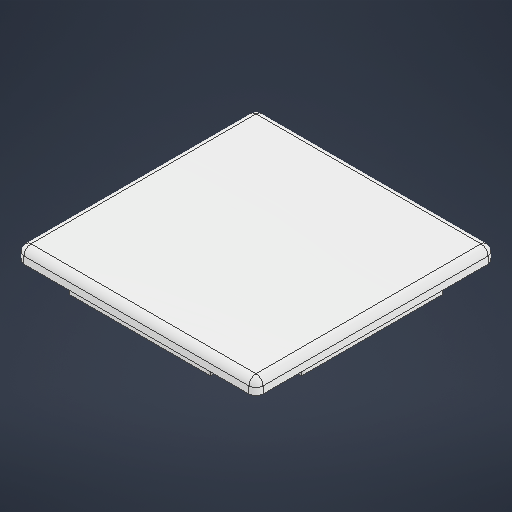
# Autodesk Inventor part: block_main
Saved by Autodesk Inventor 2025.2 (Build 292293000, 293)
## iProperties
Created: 2025-08-04
Part Number: block_main
Material: PC/ABS Plastic
Document SubType Name: Modeling
Designer: sam
Density: 1.1 g/cm^3
Appearance: Smooth - White
Author: sam
Autodesk Inventor part; units mm, degrees
ref_plane "YZ Plane" through (0, 0, 0) normal (1, 0, 0) x (0, 1, 0)
ref_plane "XZ Plane" through (0, 0, 0) normal (0, 1, 0) x (-1, 0, 0)
ref_plane "XY Plane" through (0, 0, 0) normal (0, 0, 1) x (1, 0, 0)
sketch "Sketch4" plane through (0, 0, 0) normal (0, 1, 0) x (-1, 0, 0)
  line L0 (17, 17) -> (-17, 17)
  line L1 (-17, 17) -> (-17, -17)
  line L2 (-17, -17) -> (17, -17)
  line L3 (17, -17) -> (17, 17)
  line L4 (17, 17) -> (-17, -17) construction
  line L5 (-17, 17) -> (17, -17) construction
  point P0 (0, 0)
  dimension "d52" = 34
  dimension "d53" = 34
  constraints: 12 end point, 2 midpoint, 2 parallel, 1 horizontal, 1 perpendicular
  measures "d52" distance of L2.end L1.end
  measures "d53" distance of L1.end L0.end
extrude "Extrusion5" add sketch "Sketch4" along normal blind 2
sketch "Sketch6" plane through (0, 0, 0) normal (0, -1, 0) x (1, 0, 0)
  line L0 (-16.5, -10) -> (-15.5, -10)
  line L1 (-15.5, -10) -> (-15.5, 10)
  line L2 (-15.5, 10) -> (-16.5, 10)
  line L3 (-16.5, 10) -> (-16.5, -10)
  line L4 (-15.5, -10) -> (-16.5, -10)
  line L5 (-16.5, -10) -> (-16.5, 10)
  line L6 (-16.5, 10) -> (-15.5, 10)
  line L7 (-15.5, 10) -> (-15.5, -10)
  line L8 (-10, 16.5) -> (10, 16.5)
  line L9 (10, 16.5) -> (10, 15.5)
  line L10 (10, 15.5) -> (-10, 15.5)
  line L11 (-10, 15.5) -> (-10, 16.5)
  line L12 (10, 16.5) -> (-10, 16.5)
  line L13 (-10, 16.5) -> (-10, 15.5)
  line L14 (-10, 15.5) -> (10, 15.5)
  line L15 (10, 15.5) -> (10, 16.5)
  line L16 (15.5, 10) -> (16.5, 10)
  line L17 (16.5, 10) -> (16.5, -10)
  line L18 (16.5, -10) -> (15.5, -10)
  line L19 (15.5, -10) -> (15.5, 10)
  line L20 (15.5, -10) -> (16.5, -10)
  line L21 (16.5, -10) -> (16.5, 10)
  line L22 (16.5, 10) -> (15.5, 10)
  line L23 (15.5, 10) -> (15.5, -10)
  line L24 (10, -15.5) -> (-10, -15.5)
  line L25 (-10, -15.5) -> (-10, -16.5)
  line L26 (-10, -16.5) -> (10, -16.5)
  line L27 (10, -16.5) -> (10, -15.5)
  line L28 (-10, -15.5) -> (10, -15.5)
  line L29 (10, -15.5) -> (10, -16.5)
  line L30 (10, -16.5) -> (-10, -16.5)
  line L31 (-10, -16.5) -> (-10, -15.5)
  line L32 (-17, 17) -> (-17, -17)
  line L33 (17, 17) -> (-17, 17)
  line L34 (17, -17) -> (17, 17)
  line L35 (-17, -17) -> (17, -17)
  line L36 (17, 17) -> (17, -17) projected
  line L37 (-17, -17) -> (-17, 17) projected
  line L38 (-17, 17) -> (17, 17) projected
  line L39 (17, -17) -> (-17, -17) projected
  point P0 (0, 0)
  point P1 (-16, 10)
  point P2 (-16, -10)
  point P3 (16, 10)
  point P4 (16, -10)
  point P5 (-10, -16)
  point P6 (-16, -10)
  dimension "d123" = 1
  dimension "d124" = 20
  dimension "d119" = 1
  dimension "d118" = 20
  dimension "d116" = 20
  dimension "d117" = 1
  dimension "d112" = 20
  dimension "d113" = 1
  dimension "d108" = 1
  dimension "d109" = 20
  dimension "d104" = 1
  dimension "d105" = 20
  dimension "d101" = 20
  dimension "d102" = 1
  dimension "d97" = 20
  dimension "d98" = 1
  dimension "d114" = 7
  dimension "d115" = 0.5
  dimension "d111" = 0.5
  dimension "d110" = 7
  dimension "d107" = 7
  dimension "d106" = 0.5
  dimension "d103" = 0.5
  dimension "d95" = 7
  dimension "d99" = 7
  dimension "d100" = 0.5
  dimension "d96" = 0.5
  dimension "d94" = 7
  dimension "d93" = 7
  dimension "d122" = 0.5
  dimension "d120" = 7
  dimension "d121" = 0.5
  dimension "d133" = 0
  dimension "d134" = 0
  dimension "d135" = 0
  dimension "d136" = 0
  constraints: 72 end point, 14 parallel, 7 horizontal, 7 perpendicular, 6 midpoint
  measures "d123" distance of L2.end L1.end
  measures "d124" distance of L1.end L0.end
  measures "d119" distance between parallel lines of L7 L5
  measures "d118" distance of point (-16, 10) point (-16, -10)
  measures "d116" distance of L9.end L10.end
  measures "d117" distance of L8.end L9.end
  measures "d112" distance of L14.end L13.end
  measures "d113" distance of L13.end L12.end
  measures "d108" distance of L17.end L18.end
  measures "d109" distance of L16.end L17.end
  measures "d104" distance of L22.end L21.end
  measures "d105" distance of L21.end L20.end
  measures "d101" distance of L26.end L25.end
  measures "d102" distance of L25.end L24.end
  measures "d97" distance of L29.end L30.end
  measures "d98" distance of L28.end L29.end
  measures "d114" distance between parallel lines of L32 L11
  measures "d115" distance between parallel lines of L33 L8
  measures "d111" distance between parallel lines of L33 L12
  measures "d110" distance between parallel lines of L34 L15
  measures "d107" distance between parallel lines of L33 L16
  measures "d106" distance between parallel lines of L34 L17
  measures "d103" distance between parallel lines of L34 L21
  measures "d95" distance from line of L35 point (16, -10)
  measures "d99" distance between parallel lines of L34 L27
  measures "d100" distance between parallel lines of L35 L26
  measures "d96" distance between parallel lines of L35 L30
  measures "d94" distance from line of L32 point (-10, -16)
  measures "d93" distance from line of L35 point (-16, -10)
  measures "d122" distance between parallel lines of L32 L3
  measures "d120" distance between parallel lines of L33 L6
  measures "d121" distance between parallel lines of L32 L5
  measures "d133" distance between parallel lines of L36 L34
  measures "d134" distance between parallel lines of L37 L32
  measures "d135" distance between parallel lines of L38 L33
  measures "d136" distance between parallel lines of L35 L39
extrude "Extrusion7" add sketch "Sketch6" along normal blind 1 contours L3 L2 L1 L0 | L8 L9 L10 L11 | L16 L17 L18 L19 | L27 L26 L25 L24
fillet "Fillet9" radius 1 1 edges at (17, 1, -17)
fillet "Fillet10" radius 1 1 edges at (-17, 1, -17)
fillet "Fillet11" radius 1 1 edges at (-17, 1, 17)
fillet "Fillet12" radius 1 1 edges at (17, 1, 17)
fillet "Fillet13" radius 1 8 edges at (-16.7071, 2, -16.7071) (-17, 2, 0) (-16.7071, 2, 16.7071) (0, 2, 17) (16.7071, 2, 16.7071) (17, 2, 0) (16.7071, 2, -16.7071) (0, 2, -17)
body "Solid1"
